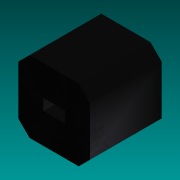
# Autodesk Inventor part: Holder
Saved by Autodesk Inventor 2015 (Build 190159000, 159)
## iProperties
Created: 2014-07-19
Part Number: Holder
Material: ABS Plastic
Document SubType Name: Modeling
Designer: Sawaiz Syed
Density: 1.06 g/cm^3
Appearance: Smooth - Black
Author: Sawaiz Syed
Autodesk Inventor part; units mm, degrees
ref_plane "YZ Plane" through (0, 0, 0) normal (1, 0, 0) x (0, 1, 0)
ref_plane "XZ Plane" through (0, 0, 0) normal (0, 1, 0) x (-1, 0, 0)
ref_plane "XY Plane" through (0, 0, 0) normal (0, 0, 1) x (1, 0, 0)
sketch "Sketch1" plane through (0, 0, 0) normal (0, 1, 0) x (-1, 0, 0)
  line L0 (0.87, -1.27) -> (-0.87, -1.27)
  line L1 (-1.27, -0.87) -> (-1.27, 0.87)
  line L2 (-0.87, 1.27) -> (0.87, 1.27)
  line L3 (1.27, 0.87) -> (1.27, -0.87)
  line L4 (1.27, -1.27) -> (-1.27, 1.27) construction
  line L5 (-1.27, -1.27) -> (1.27, 1.27) construction
  line L6 (0.381, -0.203) -> (-0.381, -0.203)
  line L7 (-0.381, -0.203) -> (-0.381, 0.203)
  line L8 (-0.381, 0.203) -> (0.381, 0.203)
  line L9 (0.381, 0.203) -> (0.381, -0.203)
  line L10 (0.381, -0.203) -> (-0.381, 0.203) construction
  line L11 (-0.381, -0.203) -> (0.381, 0.203) construction
  line L12 (0.87, -1.27) -> (1.27, -0.87)
  line L13 (-0.87, -1.27) -> (-1.27, -0.87)
  line L14 (-1.27, 0.87) -> (-0.87, 1.27)
  line L15 (0.87, 1.27) -> (1.27, 0.87)
  point P0 (0, 0)
  dimension "d0" = 2.54
  dimension "d1" = 2.54
  dimension "d2" = 0.406
  dimension "d3" = 0.762
  dimension "d4" = 0.4
  dimension "d5" = 0.4
  dimension "d6" = 0.4
  dimension "d7" = 0.4
  dimension "d8" = 0.4
  dimension "d9" = 0.4
  dimension "d10" = 0.4
  dimension "d11" = 0.4
  constraints: 32 end point, 8 point on line, 4 midpoint, 4 parallel, 2 horizontal, 2 perpendicular
  measures "d0" distance of L4.end L5.end
  measures "d1" distance of L5.start L4.end
  measures "d2" distance of L8.end L6.start
  measures "d3" distance of L7.end L8.end
  measures "d4" distance of L0.start L4.start
  measures "d5" distance of L3.end L4.start
  measures "d6" distance of L0.end L5.start
  measures "d7" distance of L1.start L5.start
  measures "d8" distance of L1.end L4.end
  measures "d9" distance of L2.start L4.end
  measures "d10" distance of L2.end L5.end
  measures "d11" distance of L3.start L5.end
extrude "Extrusion1" add sketch "Sketch1" along normal blind 2.54
equation "\"d5\" = d4"
equation "\"d6\" = d4"
equation "\"d7\" = d6"
equation "\"d8\" = d4"
equation "\"d9\" = d8"
equation "\"d10\" = d4"
equation "\"d11\" = d10"
body "Solid1"
